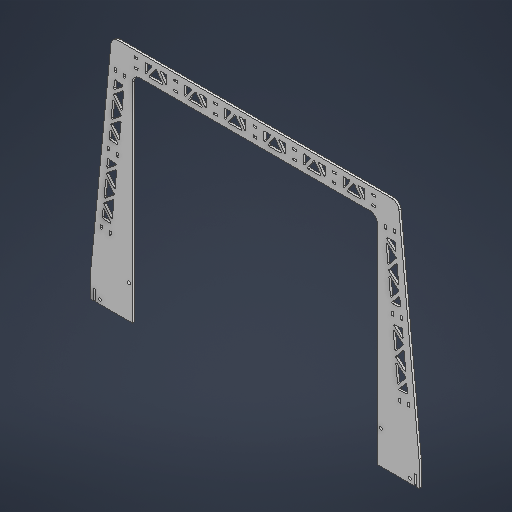
# Autodesk Inventor part: GateBrigeSideLessMaterial
Saved by Autodesk Inventor 2026 (Build 300175000, 175)
## iProperties
Created: 2025-03-30
Part Number: GateBrigeSideLessMaterial
Material: Všeobecné
Document SubType Name: Modeling
Designer: 42060
Density: 1 g/cm^3
Appearance: Výchozí
Author: 42060
Autodesk Inventor part; units mm, degrees
ref_plane "YZ Plane" through (0, 0, 0) normal (1, 0, 0) x (0, 1, 0)
ref_plane "XZ Plane" through (0, 0, 0) normal (0, 1, 0) x (-1, 0, 0)
ref_plane "XY Plane" through (0, 0, 0) normal (0, 0, 1) x (1, 0, 0)
sketch "Náčrt1" plane through (0, 0, 0) normal (0, 0, 1) x (1, 0, 0)
  line L0 (0, 0) -> (-160, 0)
  line L1 (-170, -10) -> (-170, -300)
  line L2 (-228, -300) -> (-228, -265.3)
  line L3 (-190.0475, 30) -> (0, 30)
  line L4 (0, 30) -> (0, 0)
  line L5 (-203.7, -249) -> (-170, -249)
  line L6 (-170, -249) -> (-170, -299)
  line L7 (-170, -299) -> (-220, -299)
  line L8 (-220, -299) -> (-220, -265.3)
  line L9 (-220, -265.3) -> (-203.7, -249)
  line L10 (-220, -299) -> (-170, -249) construction
  circle A0 centre (-215, -294) radius 2.1
  circle A1 centre (-175, -254) radius 2.1
  arc A2 (-160, 0) -> (-170, -10) centre (-160, -10) ccw
  line L11 (-200, 20.9734) -> (-228, -265.3)
  arc A3 (-190.0475, 30) -> (-200, 20.9734) centre (-190.0475, 20) ccw
  line L12 (-224, -300) -> (-224, -285)
  line L13 (-224, -285) -> (-221, -285)
  line L14 (-221, -285) -> (-221, -300)
  line L15 (-170, -300) -> (-221, -300)
  line L16 (-224, -300) -> (-228, -300)
  line L17 (0, 0) -> (160, 0)
  line L18 (170, -10) -> (170, -300)
  line L19 (228, -300) -> (228, -265.3)
  line L20 (190.0475, 30) -> (0, 30)
  line L21 (203.7, -249) -> (170, -249)
  line L22 (170, -249) -> (170, -299)
  line L23 (170, -299) -> (220, -299)
  line L24 (220, -299) -> (220, -265.3)
  line L25 (220, -265.3) -> (203.7, -249)
  line L26 (220, -299) -> (170, -249) construction
  circle A4 centre (215, -294) radius 2.1
  circle A5 centre (175, -254) radius 2.1
  arc A6 (170, -10) -> (160, 0) centre (160, -10) ccw
  line L27 (200, 20.9734) -> (228, -265.3)
  arc A7 (200, 20.9734) -> (190.0475, 30) centre (190.0475, 20) ccw
  line L28 (224, -300) -> (224, -285)
  line L29 (224, -285) -> (221, -285)
  line L30 (221, -285) -> (221, -300)
  line L31 (170, -300) -> (221, -300)
  line L32 (224, -300) -> (228, -300)
  line L33 (-36.6095, 9.0611) -> (-28.3278, 21.2788)
  line L34 (-26.6722, 21.2788) -> (-18.3905, 9.0611)
  line L35 (-19.2183, 7.5) -> (-35.7817, 7.5)
  line L36 (-21.6095, 20.9389) -> (-14.3278, 10.1964)
  line L37 (-12.5, 10.7575) -> (-12.5, 21.5)
  line L38 (-13.5, 22.5) -> (-20.7817, 22.5)
  line L39 (-33.3905, 20.9389) -> (-40.6722, 10.1964)
  line L40 (-42.5, 10.7575) -> (-42.5, 21.5)
  line L41 (-41.5, 22.5) -> (-34.2183, 22.5)
  line L42 (-55, 15) -> (0, 15) construction
  arc A8 (-41.5, 22.5) -> (-42.5, 21.5) centre (-41.5, 21.5) ccw
  arc A9 (-33.3905, 20.9389) -> (-34.2183, 22.5) centre (-34.2183, 21.5) ccw
  arc A10 (-42.5, 10.7575) -> (-40.6722, 10.1964) centre (-41.5, 10.7575) ccw
  arc A11 (-36.6095, 9.0611) -> (-35.7817, 7.5) centre (-35.7817, 8.5) ccw
  arc A12 (-19.2183, 7.5) -> (-18.3905, 9.0611) centre (-19.2183, 8.5) ccw
  arc A13 (-26.6722, 21.2788) -> (-28.3278, 21.2788) centre (-27.5, 20.7178) ccw
  arc A14 (-20.7817, 22.5) -> (-21.6095, 20.9389) centre (-20.7817, 21.5) ccw
  arc A15 (-12.5, 21.5) -> (-13.5, 22.5) centre (-13.5, 21.5) ccw
  arc A16 (-14.3278, 10.1964) -> (-12.5, 10.7575) centre (-13.5, 10.7575) ccw
  arc A17 (-81.6722, 21.2788) -> (-83.3278, 21.2788) centre (-82.5, 20.7178) ccw
  line L43 (-91.6095, 9.0611) -> (-83.3278, 21.2788)
  line L44 (-68.5, 22.5) -> (-75.7817, 22.5)
  arc A18 (-67.5, 21.5) -> (-68.5, 22.5) centre (-68.5, 21.5) ccw
  line L45 (-81.6722, 21.2788) -> (-73.3905, 9.0611)
  arc A19 (-74.2183, 7.5) -> (-73.3905, 9.0611) centre (-74.2183, 8.5) ccw
  line L46 (-76.6095, 20.9389) -> (-69.3278, 10.1964)
  line L47 (-74.2183, 7.5) -> (-90.7817, 7.5)
  arc A20 (-69.3278, 10.1964) -> (-67.5, 10.7575) centre (-68.5, 10.7575) ccw
  line L48 (-110, 15) -> (-55, 15) construction
  arc A21 (-96.5, 22.5) -> (-97.5, 21.5) centre (-96.5, 21.5) ccw
  arc A22 (-97.5, 10.7575) -> (-95.6722, 10.1964) centre (-96.5, 10.7575) ccw
  arc A23 (-91.6095, 9.0611) -> (-90.7817, 7.5) centre (-90.7817, 8.5) ccw
  arc A24 (-88.3905, 20.9389) -> (-89.2183, 22.5) centre (-89.2183, 21.5) ccw
  line L49 (-67.5, 10.7575) -> (-67.5, 21.5)
  arc A25 (-75.7817, 22.5) -> (-76.6095, 20.9389) centre (-75.7817, 21.5) ccw
  line L50 (-96.5, 22.5) -> (-89.2183, 22.5)
  line L51 (-88.3905, 20.9389) -> (-95.6722, 10.1964)
  line L52 (-97.5, 10.7575) -> (-97.5, 21.5)
  arc A26 (-136.6722, 21.2788) -> (-138.3278, 21.2788) centre (-137.5, 20.7178) ccw
  line L53 (-146.6095, 9.0611) -> (-138.3278, 21.2788)
  line L54 (-123.5, 22.5) -> (-130.7817, 22.5)
  arc A27 (-122.5, 21.5) -> (-123.5, 22.5) centre (-123.5, 21.5) ccw
  line L55 (-136.6722, 21.2788) -> (-128.3905, 9.0611)
  arc A28 (-129.2183, 7.5) -> (-128.3905, 9.0611) centre (-129.2183, 8.5) ccw
  line L56 (-131.6095, 20.9389) -> (-124.3278, 10.1964)
  line L57 (-129.2183, 7.5) -> (-145.7817, 7.5)
  arc A29 (-124.3278, 10.1964) -> (-122.5, 10.7575) centre (-123.5, 10.7575) ccw
  line L58 (-165, 15) -> (-110, 15) construction
  arc A30 (-151.5, 22.5) -> (-152.5, 21.5) centre (-151.5, 21.5) ccw
  arc A31 (-152.5, 10.7575) -> (-150.6722, 10.1964) centre (-151.5, 10.7575) ccw
  arc A32 (-146.6095, 9.0611) -> (-145.7817, 7.5) centre (-145.7817, 8.5) ccw
  arc A33 (-143.3905, 20.9389) -> (-144.2183, 22.5) centre (-144.2183, 21.5) ccw
  line L59 (-122.5, 10.7575) -> (-122.5, 21.5)
  arc A34 (-130.7817, 22.5) -> (-131.6095, 20.9389) centre (-130.7817, 21.5) ccw
  line L60 (-151.5, 22.5) -> (-144.2183, 22.5)
  line L61 (-143.3905, 20.9389) -> (-150.6722, 10.1964)
  line L62 (-152.5, 10.7575) -> (-152.5, 21.5)
  line L63 (-193.8722, -19.4692) -> (-183.9904, -20.4358)
  line L64 (-183.4529, -22.2036) -> (-194.3012, -31.1189)
  line L65 (-195.9313, -30.2489) -> (-194.9648, -20.3672)
  line L66 (-182.3734, -28.7035) -> (-184.5011, -50.4576)
  line L67 (-186.2689, -50.9951) -> (-196.0821, -39.0542)
  line L68 (-195.9444, -37.6468) -> (-184.0035, -27.8336)
  line L69 (-195.7348, -45.7768) -> (-185.9217, -57.7177)
  line L70 (-186.0594, -59.1252) -> (-198.0002, -68.9384)
  line L71 (-199.6304, -68.0685) -> (-197.5027, -46.3144)
  line L72 (-187.7026, -65.6531) -> (-199.6435, -75.4663)
  line L73 (-199.7812, -76.8738) -> (-189.968, -88.8147)
  line L74 (-188.2002, -88.2771) -> (-186.0724, -66.523)
  line L75 (-199.4339, -83.5964) -> (-190.5187, -94.4447)
  line L76 (-191.3886, -96.0748) -> (-201.2704, -95.1083)
  line L77 (-202.1683, -94.0157) -> (-201.2018, -84.1339)
  line L78 (-188.9313, -19.9525) -> (-188.0066, -10.4976) construction
  arc A35 (-193.8722, -19.4692) -> (-194.9648, -20.3672) centre (-193.9696, -20.4645) ccw
  arc A36 (-183.4529, -22.2036) -> (-183.9904, -20.4358) centre (-184.0878, -21.431) ccw
  arc A37 (-195.9313, -30.2489) -> (-194.3012, -31.1189) centre (-194.9361, -30.3463) ccw
  arc A38 (-195.9444, -37.6468) -> (-196.0821, -39.0542) centre (-195.3095, -38.4193) ccw
  arc A39 (-186.2689, -50.9951) -> (-184.5011, -50.4576) centre (-185.4963, -50.3602) ccw
  arc A40 (-182.3734, -28.7035) -> (-184.0035, -27.8336) centre (-183.3686, -28.6062) ccw
  arc A41 (-195.7348, -45.7768) -> (-197.5027, -46.3144) centre (-196.5074, -46.4117) ccw
  arc A42 (-186.0594, -59.1252) -> (-185.9217, -57.7177) centre (-186.6943, -58.3526) ccw
  arc A43 (-199.6304, -68.0685) -> (-198.0002, -68.9384) centre (-198.6352, -68.1658) ccw
  arc A44 (-199.6435, -75.4663) -> (-199.7812, -76.8738) centre (-199.0086, -76.2389) ccw
  arc A45 (-189.968, -88.8147) -> (-188.2002, -88.2771) centre (-189.1954, -88.1798) ccw
  arc A46 (-186.0724, -66.523) -> (-187.7026, -65.6531) centre (-187.0677, -66.4257) ccw
  arc A47 (-199.4339, -83.5964) -> (-201.2018, -84.1339) centre (-200.2065, -84.2313) ccw
  arc A48 (-202.1683, -94.0157) -> (-201.2704, -95.1083) centre (-201.173, -94.1131) ccw
  arc A49 (-191.3886, -96.0748) -> (-190.5187, -94.4447) centre (-191.2912, -95.0796) ccw
  arc A50 (-211.9027, -193.5408) -> (-211.0048, -194.6334) centre (-210.9074, -193.6381) ccw
  line L79 (-201.123, -195.5999) -> (-211.0048, -194.6334)
  arc A51 (-201.123, -195.5999) -> (-200.2531, -193.9697) centre (-201.0257, -194.6047) ccw
  arc A52 (-199.7024, -188.3398) -> (-197.9346, -187.8022) centre (-198.9298, -187.7048) ccw
  line L80 (-209.1683, -183.1214) -> (-200.2531, -193.9697)
  line L81 (-211.9027, -193.5408) -> (-210.9362, -183.659)
  arc A53 (-209.1683, -183.1214) -> (-210.9362, -183.659) centre (-209.9409, -183.7564) ccw
  line L82 (-197.437, -165.1782) -> (-209.3779, -174.9914)
  line L83 (-209.5156, -176.3989) -> (-199.7024, -188.3398)
  line L84 (-197.9346, -187.8022) -> (-195.8068, -166.0481)
  arc A54 (-209.3779, -174.9914) -> (-209.5156, -176.3989) centre (-208.743, -175.7639) ccw
  arc A55 (-209.3648, -167.5935) -> (-207.7347, -168.4635) centre (-208.3696, -167.6909) ccw
  arc A56 (-195.8068, -166.0481) -> (-197.437, -165.1782) centre (-196.8021, -165.9508) ccw
  line L85 (-205.4693, -145.3019) -> (-195.6561, -157.2428)
  arc A57 (-195.7938, -158.6503) -> (-195.6561, -157.2428) centre (-196.4287, -157.8777) ccw
  line L86 (-209.3648, -167.5935) -> (-207.2371, -145.8395)
  line L87 (-195.7938, -158.6503) -> (-207.7347, -168.4635)
  arc A58 (-196.0033, -150.5202) -> (-194.2355, -149.9827) centre (-195.2308, -149.8853) ccw
  arc A59 (-205.4693, -145.3019) -> (-207.2371, -145.8395) centre (-206.2418, -145.9368) ccw
  line L88 (-196.0033, -150.5202) -> (-205.8165, -138.5793)
  arc A60 (-205.6788, -137.1718) -> (-205.8165, -138.5793) centre (-205.0439, -137.9444) ccw
  arc A61 (-205.6657, -129.774) -> (-204.0356, -130.6439) centre (-204.6705, -129.8714) ccw
  line L89 (-192.1078, -128.2286) -> (-194.2355, -149.9827)
  line L90 (-205.6788, -137.1718) -> (-193.7379, -127.3587)
  arc A62 (-192.1078, -128.2286) -> (-193.7379, -127.3587) centre (-193.103, -128.1312) ccw
  arc A63 (-193.1873, -121.7287) -> (-193.7248, -119.9608) centre (-193.8222, -120.9561) ccw
  line L91 (-198.6657, -119.4776) -> (-197.741, -110.0227) construction
  line L92 (-203.6066, -118.9943) -> (-193.7248, -119.9608)
  arc A64 (-203.6066, -118.9943) -> (-204.6992, -119.8922) centre (-203.704, -119.9896) ccw
  line L93 (-193.1873, -121.7287) -> (-204.0356, -130.6439)
  line L94 (-205.6657, -129.774) -> (-204.6992, -119.8922)
  line L95 (36.6095, 9.0611) -> (28.3278, 21.2788)
  line L96 (26.6722, 21.2788) -> (18.3905, 9.0611)
  line L97 (19.2183, 7.5) -> (35.7817, 7.5)
  line L98 (21.6095, 20.9389) -> (14.3278, 10.1964)
  line L99 (12.5, 10.7575) -> (12.5, 21.5)
  line L100 (13.5, 22.5) -> (20.7817, 22.5)
  line L101 (33.3905, 20.9389) -> (40.6722, 10.1964)
  line L102 (42.5, 10.7575) -> (42.5, 21.5)
  line L103 (41.5, 22.5) -> (34.2183, 22.5)
  line L104 (55, 15) -> (0, 15) construction
  arc A65 (42.5, 21.5) -> (41.5, 22.5) centre (41.5, 21.5) ccw
  arc A66 (34.2183, 22.5) -> (33.3905, 20.9389) centre (34.2183, 21.5) ccw
  arc A67 (40.6722, 10.1964) -> (42.5, 10.7575) centre (41.5, 10.7575) ccw
  arc A68 (35.7817, 7.5) -> (36.6095, 9.0611) centre (35.7817, 8.5) ccw
  arc A69 (18.3905, 9.0611) -> (19.2183, 7.5) centre (19.2183, 8.5) ccw
  arc A70 (28.3278, 21.2788) -> (26.6722, 21.2788) centre (27.5, 20.7178) ccw
  arc A71 (21.6095, 20.9389) -> (20.7817, 22.5) centre (20.7817, 21.5) ccw
  arc A72 (13.5, 22.5) -> (12.5, 21.5) centre (13.5, 21.5) ccw
  arc A73 (12.5, 10.7575) -> (14.3278, 10.1964) centre (13.5, 10.7575) ccw
  line L105 (67.5, 10.7575) -> (67.5, 21.5)
  line L106 (96.5, 22.5) -> (89.2183, 22.5)
  arc A74 (97.5, 21.5) -> (96.5, 22.5) centre (96.5, 21.5) ccw
  line L107 (97.5, 10.7575) -> (97.5, 21.5)
  arc A75 (95.6722, 10.1964) -> (97.5, 10.7575) centre (96.5, 10.7575) ccw
  arc A76 (67.5, 10.7575) -> (69.3278, 10.1964) centre (68.5, 10.7575) ccw
  arc A77 (68.5, 22.5) -> (67.5, 21.5) centre (68.5, 21.5) ccw
  arc A78 (89.2183, 22.5) -> (88.3905, 20.9389) centre (89.2183, 21.5) ccw
  arc A79 (83.3278, 21.2788) -> (81.6722, 21.2788) centre (82.5, 20.7178) ccw
  line L108 (88.3905, 20.9389) -> (95.6722, 10.1964)
  line L109 (91.6095, 9.0611) -> (83.3278, 21.2788)
  arc A80 (76.6095, 20.9389) -> (75.7817, 22.5) centre (75.7817, 21.5) ccw
  arc A81 (90.7817, 7.5) -> (91.6095, 9.0611) centre (90.7817, 8.5) ccw
  line L110 (110, 15) -> (55, 15) construction
  line L111 (68.5, 22.5) -> (75.7817, 22.5)
  line L112 (76.6095, 20.9389) -> (69.3278, 10.1964)
  line L113 (81.6722, 21.2788) -> (73.3905, 9.0611)
  arc A82 (73.3905, 9.0611) -> (74.2183, 7.5) centre (74.2183, 8.5) ccw
  line L114 (74.2183, 7.5) -> (90.7817, 7.5)
  line L115 (122.5, 10.7575) -> (122.5, 21.5)
  line L116 (151.5, 22.5) -> (144.2183, 22.5)
  arc A83 (152.5, 21.5) -> (151.5, 22.5) centre (151.5, 21.5) ccw
  line L117 (152.5, 10.7575) -> (152.5, 21.5)
  arc A84 (150.6722, 10.1964) -> (152.5, 10.7575) centre (151.5, 10.7575) ccw
  arc A85 (122.5, 10.7575) -> (124.3278, 10.1964) centre (123.5, 10.7575) ccw
  arc A86 (123.5, 22.5) -> (122.5, 21.5) centre (123.5, 21.5) ccw
  arc A87 (144.2183, 22.5) -> (143.3905, 20.9389) centre (144.2183, 21.5) ccw
  arc A88 (138.3278, 21.2788) -> (136.6722, 21.2788) centre (137.5, 20.7178) ccw
  line L118 (143.3905, 20.9389) -> (150.6722, 10.1964)
  line L119 (146.6095, 9.0611) -> (138.3278, 21.2788)
  arc A89 (131.6095, 20.9389) -> (130.7817, 22.5) centre (130.7817, 21.5) ccw
  arc A90 (145.7817, 7.5) -> (146.6095, 9.0611) centre (145.7817, 8.5) ccw
  line L120 (165, 15) -> (110, 15) construction
  line L121 (123.5, 22.5) -> (130.7817, 22.5)
  line L122 (131.6095, 20.9389) -> (124.3278, 10.1964)
  line L123 (136.6722, 21.2788) -> (128.3905, 9.0611)
  arc A91 (128.3905, 9.0611) -> (129.2183, 7.5) centre (129.2183, 8.5) ccw
  line L124 (129.2183, 7.5) -> (145.7817, 7.5)
  line L125 (193.8722, -19.4692) -> (183.9904, -20.4358)
  line L126 (183.4529, -22.2036) -> (194.3012, -31.1189)
  line L127 (195.9313, -30.2489) -> (194.9648, -20.3672)
  line L128 (182.3734, -28.7035) -> (184.5011, -50.4576)
  line L129 (186.2689, -50.9951) -> (196.0821, -39.0542)
  line L130 (195.9444, -37.6468) -> (184.0035, -27.8336)
  line L131 (195.7348, -45.7768) -> (185.9217, -57.7177)
  line L132 (186.0594, -59.1252) -> (198.0002, -68.9384)
  line L133 (199.6304, -68.0685) -> (197.5027, -46.3144)
  line L134 (187.7026, -65.6531) -> (199.6435, -75.4663)
  line L135 (199.7812, -76.8738) -> (189.968, -88.8147)
  line L136 (188.2002, -88.2771) -> (186.0724, -66.523)
  line L137 (199.4339, -83.5964) -> (190.5187, -94.4447)
  line L138 (191.3886, -96.0748) -> (201.2704, -95.1083)
  line L139 (202.1683, -94.0157) -> (201.2018, -84.1339)
  arc A92 (194.9648, -20.3672) -> (193.8722, -19.4692) centre (193.9696, -20.4645) ccw
  arc A93 (183.9904, -20.4358) -> (183.4529, -22.2036) centre (184.0878, -21.431) ccw
  arc A94 (194.3012, -31.1189) -> (195.9313, -30.2489) centre (194.9361, -30.3463) ccw
  arc A95 (196.0821, -39.0542) -> (195.9444, -37.6468) centre (195.3095, -38.4193) ccw
  arc A96 (184.5011, -50.4576) -> (186.2689, -50.9951) centre (185.4963, -50.3602) ccw
  arc A97 (184.0035, -27.8336) -> (182.3734, -28.7035) centre (183.3686, -28.6062) ccw
  arc A98 (197.5027, -46.3144) -> (195.7348, -45.7768) centre (196.5074, -46.4117) ccw
  arc A99 (185.9217, -57.7177) -> (186.0594, -59.1252) centre (186.6943, -58.3526) ccw
  arc A100 (198.0002, -68.9384) -> (199.6304, -68.0685) centre (198.6352, -68.1658) ccw
  arc A101 (199.7812, -76.8738) -> (199.6435, -75.4663) centre (199.0086, -76.2389) ccw
  arc A102 (188.2002, -88.2771) -> (189.968, -88.8147) centre (189.1954, -88.1798) ccw
  arc A103 (187.7026, -65.6531) -> (186.0724, -66.523) centre (187.0677, -66.4257) ccw
  arc A104 (201.2018, -84.1339) -> (199.4339, -83.5964) centre (200.2065, -84.2313) ccw
  arc A105 (201.2704, -95.1083) -> (202.1683, -94.0157) centre (201.173, -94.1131) ccw
  arc A106 (190.5187, -94.4447) -> (191.3886, -96.0748) centre (191.2912, -95.0796) ccw
  arc A107 (193.7248, -119.9608) -> (193.1873, -121.7287) centre (193.8222, -120.9561) ccw
  arc A108 (193.7379, -127.3587) -> (192.1078, -128.2286) centre (193.103, -128.1312) ccw
  line L140 (203.6066, -118.9943) -> (193.7248, -119.9608)
  line L141 (193.1873, -121.7287) -> (204.0356, -130.6439)
  line L142 (205.6657, -129.774) -> (204.6992, -119.8922)
  line L143 (205.6788, -137.1718) -> (193.7379, -127.3587)
  arc A109 (204.6992, -119.8922) -> (203.6066, -118.9943) centre (203.704, -119.9896) ccw
  arc A110 (204.0356, -130.6439) -> (205.6657, -129.774) centre (204.6705, -129.8714) ccw
  line L144 (192.1078, -128.2286) -> (194.2355, -149.9827)
  arc A111 (207.2371, -145.8395) -> (205.4693, -145.3019) centre (206.2418, -145.9368) ccw
  line L145 (196.0033, -150.5202) -> (205.8165, -138.5793)
  arc A112 (205.8165, -138.5793) -> (205.6788, -137.1718) centre (205.0439, -137.9444) ccw
  arc A113 (194.2355, -149.9827) -> (196.0033, -150.5202) centre (195.2308, -149.8853) ccw
  line L146 (205.4693, -145.3019) -> (195.6561, -157.2428)
  arc A114 (195.6561, -157.2428) -> (195.7938, -158.6503) centre (196.4287, -157.8777) ccw
  arc A115 (197.437, -165.1782) -> (195.8068, -166.0481) centre (196.8021, -165.9508) ccw
  line L147 (195.7938, -158.6503) -> (207.7347, -168.4635)
  arc A116 (207.7347, -168.4635) -> (209.3648, -167.5935) centre (208.3696, -167.6909) ccw
  line L148 (209.3648, -167.5935) -> (207.2371, -145.8395)
  arc A117 (200.2531, -193.9697) -> (201.123, -195.5999) centre (201.0257, -194.6047) ccw
  arc A118 (211.0048, -194.6334) -> (211.9027, -193.5408) centre (210.9074, -193.6381) ccw
  arc A119 (197.9346, -187.8022) -> (199.7024, -188.3398) centre (198.9298, -187.7048) ccw
  line L149 (211.9027, -193.5408) -> (210.9362, -183.659)
  line L150 (209.1683, -183.1214) -> (200.2531, -193.9697)
  arc A120 (210.9362, -183.659) -> (209.1683, -183.1214) centre (209.9409, -183.7564) ccw
  line L151 (209.5156, -176.3989) -> (199.7024, -188.3398)
  arc A121 (209.5156, -176.3989) -> (209.3779, -174.9914) centre (208.743, -175.7639) ccw
  line L152 (197.9346, -187.8022) -> (195.8068, -166.0481)
  line L153 (197.437, -165.1782) -> (209.3779, -174.9914)
  line L154 (201.123, -195.5999) -> (211.0048, -194.6334)
  line L155 (-2.5, 10) -> (2.5, 10)
  line L156 (2.5, 10) -> (2.5, 7.5)
  line L157 (2.5, 7.5) -> (-2.5, 7.5)
  line L158 (-2.5, 7.5) -> (-2.5, 10)
  line L159 (-2.5, 22.5) -> (2.5, 22.5)
  line L160 (2.5, 22.5) -> (2.5, 20)
  line L161 (2.5, 20) -> (-2.5, 20)
  line L162 (-2.5, 20) -> (-2.5, 22.5)
  line L163 (0, 20) -> (0, 10) construction
  line L164 (-42.5, 10.7575) -> (-42.5, 7.5) construction
  line L165 (-42.5, 7.5) -> (-40.6722, 10.1964) construction
  line L166 (-27.5, 22.5) -> (-27.5, 7.5) construction
  line L167 (-52.5, 10) -> (-52.5, 7.5)
  line L168 (-57.5, 10) -> (-52.5, 10)
  line L169 (-52.5, 7.5) -> (-57.5, 7.5)
  line L170 (-57.5, 7.5) -> (-57.5, 10)
  line L171 (-57.5, 22.5) -> (-52.5, 22.5)
  line L172 (-52.5, 20) -> (-57.5, 20)
  line L173 (-57.5, 20) -> (-57.5, 22.5)
  line L174 (-52.5, 22.5) -> (-52.5, 20)
  line L175 (-107.5, 10) -> (-107.5, 7.5)
  line L176 (-112.5, 10) -> (-107.5, 10)
  line L177 (-107.5, 7.5) -> (-112.5, 7.5)
  line L178 (-112.5, 7.5) -> (-112.5, 10)
  line L179 (-112.5, 22.5) -> (-107.5, 22.5)
  line L180 (-107.5, 20) -> (-112.5, 20)
  line L181 (-112.5, 20) -> (-112.5, 22.5)
  line L182 (-107.5, 22.5) -> (-107.5, 20)
  line L183 (-162.5, 10) -> (-162.5, 7.5)
  line L184 (-167.5, 10) -> (-162.5, 10)
  line L185 (-162.5, 7.5) -> (-167.5, 7.5)
  line L186 (-167.5, 7.5) -> (-167.5, 10)
  line L187 (-167.5, 22.5) -> (-162.5, 22.5)
  line L188 (-162.5, 20) -> (-167.5, 20)
  line L189 (-167.5, 20) -> (-167.5, 22.5)
  line L190 (-162.5, 22.5) -> (-162.5, 20)
  line L191 (52.5, 20) -> (52.5, 22.5)
  line L192 (57.5, 20) -> (52.5, 20)
  line L193 (57.5, 22.5) -> (57.5, 20)
  line L194 (52.5, 22.5) -> (57.5, 22.5)
  line L195 (57.5, 10) -> (57.5, 7.5)
  line L196 (52.5, 10) -> (57.5, 10)
  line L197 (57.5, 7.5) -> (52.5, 7.5)
  line L198 (52.5, 7.5) -> (52.5, 10)
  line L199 (107.5, 20) -> (107.5, 22.5)
  line L200 (112.5, 20) -> (107.5, 20)
  line L201 (112.5, 22.5) -> (112.5, 20)
  line L202 (107.5, 22.5) -> (112.5, 22.5)
  line L203 (112.5, 10) -> (112.5, 7.5)
  line L204 (107.5, 10) -> (112.5, 10)
  line L205 (112.5, 7.5) -> (107.5, 7.5)
  line L206 (107.5, 7.5) -> (107.5, 10)
  line L207 (162.5, 20) -> (162.5, 22.5)
  line L208 (167.5, 20) -> (162.5, 20)
  line L209 (167.5, 22.5) -> (167.5, 20)
  line L210 (162.5, 22.5) -> (167.5, 22.5)
  line L211 (167.5, 10) -> (167.5, 7.5)
  line L212 (162.5, 10) -> (167.5, 10)
  line L213 (167.5, 7.5) -> (162.5, 7.5)
  line L214 (162.5, 7.5) -> (162.5, 10)
  line L215 (-194.9842, -4.7913) -> (-192.4961, -5.0347)
  line L216 (-192.4961, -5.0347) -> (-192.9828, -10.0109)
  line L217 (-192.9828, -10.0109) -> (-195.4709, -9.7675)
  line L218 (-195.4709, -9.7675) -> (-194.9842, -4.7913)
  line L219 (-182.5436, -6.0081) -> (-180.0555, -6.2515)
  line L220 (-180.0555, -6.2515) -> (-180.5422, -11.2277)
  line L221 (-180.5422, -11.2277) -> (-183.0303, -10.9843)
  line L222 (-183.0303, -10.9843) -> (-182.5436, -6.0081)
  line L223 (-192.9828, -10.0109) -> (-183.0303, -10.9843) construction
  line L224 (-205.2054, -109.2926) -> (-204.7186, -104.3164)
  line L225 (-202.2305, -104.5597) -> (-202.7172, -109.536)
  line L226 (-202.7172, -109.536) -> (-205.2054, -109.2926)
  line L227 (-204.7186, -104.3164) -> (-202.2305, -104.5597)
  line L228 (-192.7647, -110.5094) -> (-192.278, -105.5332)
  line L229 (-190.2766, -110.7528) -> (-192.7647, -110.5094)
  line L230 (-189.7899, -105.7765) -> (-190.2766, -110.7528)
  line L231 (-192.278, -105.5332) -> (-189.7899, -105.7765)
  line L232 (-202.7172, -109.536) -> (-192.7647, -110.5094) construction
  line L233 (-202.2305, -104.5597) -> (-192.278, -105.5332) construction
  line L234 (-197.3029, -105.5441) -> (-196.3295, -95.5916) construction
  line L235 (-214.9398, -208.8177) -> (-214.453, -203.8414)
  line L236 (-211.9649, -204.0848) -> (-212.4516, -209.0611)
  line L237 (-212.4516, -209.0611) -> (-214.9398, -208.8177)
  line L238 (-214.453, -203.8414) -> (-211.9649, -204.0848)
  line L239 (-202.4991, -210.0345) -> (-202.0124, -205.0582)
  line L240 (-200.011, -210.2779) -> (-202.4991, -210.0345)
  line L241 (-199.5243, -205.3016) -> (-200.011, -210.2779)
  line L242 (-202.0124, -205.0582) -> (-199.5243, -205.3016)
  line L243 (-212.4516, -209.0611) -> (-202.4991, -210.0345) construction
  line L244 (194.9842, -4.7913) -> (192.4961, -5.0347)
  line L245 (192.4961, -5.0347) -> (192.9828, -10.0109)
  line L246 (192.9828, -10.0109) -> (195.4709, -9.7675)
  line L247 (195.4709, -9.7675) -> (194.9842, -4.7913)
  line L248 (182.5436, -6.0081) -> (180.0555, -6.2515)
  line L249 (180.0555, -6.2515) -> (180.5422, -11.2277)
  line L250 (180.5422, -11.2277) -> (183.0303, -10.9843)
  line L251 (183.0303, -10.9843) -> (182.5436, -6.0081)
  line L252 (205.2054, -109.2926) -> (204.7186, -104.3164)
  line L253 (202.2305, -104.5597) -> (202.7172, -109.536)
  line L254 (202.7172, -109.536) -> (205.2054, -109.2926)
  line L255 (204.7186, -104.3164) -> (202.2305, -104.5597)
  line L256 (192.7647, -110.5094) -> (192.278, -105.5332)
  line L257 (190.2766, -110.7528) -> (192.7647, -110.5094)
  line L258 (189.7899, -105.7765) -> (190.2766, -110.7528)
  line L259 (192.278, -105.5332) -> (189.7899, -105.7765)
  line L260 (214.9398, -208.8177) -> (214.453, -203.8414)
  line L261 (211.9649, -204.0848) -> (212.4516, -209.0611)
  line L262 (212.4516, -209.0611) -> (214.9398, -208.8177)
  line L263 (214.453, -203.8414) -> (211.9649, -204.0848)
  line L264 (202.4991, -210.0345) -> (202.0124, -205.0582)
  line L265 (200.011, -210.2779) -> (202.4991, -210.0345)
  line L266 (199.5243, -205.3016) -> (200.011, -210.2779)
  line L267 (202.0124, -205.0582) -> (199.5243, -205.3016)
  line L268 (-188.0066, -10.4976) -> (-187.9579, -10) construction
  point P0 (-12.5, 7.5)
  point P1 (-32.3323, 22.5)
  point P2 (-42.5, 22.5)
  point P3 (-27.5, 15)
  point P4 (-12.5, 16.1288)
  point P5 (-82.5, 22.5)
  point P6 (-82.5, 15)
  point P7 (-82.5, 7.5)
  point P8 (-87.3323, 22.5)
  point P9 (-97.5, 22.5)
  point P10 (-67.5, 7.5)
  point P11 (-67.5, 16.1288)
  point P12 (-137.5, 22.5)
  point P13 (-137.5, 15)
  point P14 (-137.5, 7.5)
  point P15 (-142.3323, 22.5)
  point P16 (-152.5, 22.5)
  point P17 (-122.5, 7.5)
  point P18 (-122.5, 16.1288)
  point P19 (-194.8675, -19.3719)
  point P20 (-181.5877, -20.6708)
  point P21 (-196.1663, -32.6517)
  point P22 (-182.1384, -26.3008)
  point P23 (-184.7361, -52.8603)
  point P24 (-196.717, -38.2817)
  point P25 (-197.2677, -43.9117)
  point P26 (-185.2868, -58.4903)
  point P27 (-199.8654, -70.4712)
  point P28 (-185.8374, -64.1203)
  point P29 (-200.4161, -76.1012)
  point P30 (-188.4352, -90.6798)
  point P31 (-200.9667, -81.7312)
  point P32 (-188.9858, -96.3098)
  point P33 (-202.2656, -95.011)
  point P34 (-212, -194.536)
  point P35 (-198.7203, -195.8349)
  point P36 (-198.1696, -190.2049)
  point P37 (-210.7012, -181.2563)
  point P38 (-210.1505, -175.6263)
  point P39 (-209.5998, -169.9963)
  point P40 (-195.5718, -163.6454)
  point P41 (-195.0212, -158.0154)
  point P42 (-194.4705, -152.3854)
  point P43 (-207.0021, -143.4367)
  point P44 (-206.4514, -137.8067)
  point P45 (-205.9008, -132.1768)
  point P46 (-191.8728, -125.8258)
  point P47 (-191.3221, -120.1959)
  point P48 (-204.6019, -118.897)
  point P49 (27.5, 22.5)
  point P50 (12.5, 7.5)
  point P51 (32.3323, 22.5)
  point P52 (42.5, 22.5)
  point P53 (27.5, 7.5)
  point P54 (27.5, 15)
  point P55 (12.5, 16.1288)
  point P56 (67.5, 7.5)
  point P57 (67.5, 16.1288)
  point P58 (82.5, 22.5)
  point P59 (87.3323, 22.5)
  point P60 (97.5, 22.5)
  point P61 (82.5, 15)
  point P62 (82.5, 7.5)
  point P63 (122.5, 7.5)
  point P64 (122.5, 16.1288)
  point P65 (137.5, 22.5)
  point P66 (142.3323, 22.5)
  point P67 (152.5, 22.5)
  point P68 (137.5, 15)
  point P69 (137.5, 7.5)
  point P70 (194.8675, -19.3719)
  point P71 (181.5877, -20.6708)
  point P72 (196.1663, -32.6517)
  point P73 (182.1384, -26.3008)
  point P74 (184.7361, -52.8603)
  point P75 (196.717, -38.2817)
  point P76 (197.2677, -43.9117)
  point P77 (185.2868, -58.4903)
  point P78 (199.8654, -70.4712)
  point P79 (185.8374, -64.1203)
  point P80 (200.4161, -76.1012)
  point P81 (188.4352, -90.6798)
  point P82 (200.9667, -81.7312)
  point P83 (188.9858, -96.3098)
  point P84 (202.2656, -95.011)
  point P85 (188.9313, -19.9525)
  point P86 (191.3221, -120.1959)
  point P87 (191.8728, -125.8258)
  point P88 (198.6657, -119.4776)
  point P89 (204.6019, -118.897)
  point P90 (205.9008, -132.1768)
  point P91 (206.4514, -137.8067)
  point P92 (194.4705, -152.3854)
  point P93 (207.0021, -143.4367)
  point P94 (195.0212, -158.0154)
  point P95 (195.5718, -163.6454)
  point P96 (209.5998, -169.9963)
  point P97 (212, -194.536)
  point P98 (198.7203, -195.8349)
  point P99 (198.1696, -190.2049)
  point P100 (210.1505, -175.6263)
  point P101 (210.7012, -181.2563)
  point P102 (0, 15)
  point P103 (-27.5, 15)
  point P104 (-55, 10)
  point P105 (-55, 20)
  point P106 (-110, 10)
  point P107 (-110, 20)
  point P108 (-165, 10)
  point P109 (-165, 20)
  point P110 (55, 20)
  point P111 (55, 10)
  point P112 (110, 20)
  point P113 (110, 10)
  point P114 (165, 20)
  point P115 (165, 10)
  point P116 (-207.4754, -209.5478)
  point P117 (-197.2542, -105.0465)
  dimension "d0" = 50
  dimension "d1" = 50
  dimension "d3" = 33.7
  dimension "d4" = 45
  dimension "d5" = 0
  dimension "d6" = 4.2
  dimension "d7" = 5
  dimension "d8" = 5
  dimension "d10" = 170
  dimension "d12" = 30
  dimension "d14" = 10
  dimension "d16" = 15
  dimension "d17" = 1
  dimension "d18" = 3
  dimension "d19" = 1
  dimension "d20" = 4
  dimension "d21" = 300
  dimension "d22" = 30
  dimension "d46" = 4
  dimension "d47" = 4
  dimension "d50" = 15
  dimension "d51" = 30
  dimension "d52" = 1
  dimension "d55" = 55
  dimension "d63" = 4
  dimension "d64" = 4
  dimension "d65" = 4
  dimension "d66" = 4
  dimension "d67" = 1
  dimension "d70" = 100
  dimension "d77" = 55
  dimension "d84" = 100
  dimension "d91" = 2.5
  dimension "d92" = 5
  dimension "d93" = 15
  dimension "d96" = 55
  dimension "d103" = 55
  dimension "d108" = 5
  dimension "d109" = 2.5
  dimension "d110" = 7.5
  dimension "d111" = 15
  dimension "d115" = 100
  dimension "d123" = 0.5
  dimension "d124" = 0.5
  dimension "d125" = 10
  dimension "d126" = 10
  constraints: 538 end point, 236 point on circle, 227 point on line, 141 symmetric about line, 122 centre point, 52 tangent, 24 equal radius, 24 perpendicular, 20 parallel, 12 midpoint, 11 collinear, 10 coincident, 10 horizontal, 5 equal length, 4 horizontal alignment, 4 vertical alignment, 2 vertical, 579 other
  measures "d0" distance of L5.end L6.end
  measures "d1" distance of L6.end L7.end
  measures "d3" distance of L5.start L5.end
  measures "d4" angle of L5 L9
  measures "d5" distance between parallel lines of L1 L6
  measures "d6" diameter of A1
  measures "d7" distance from line of L5 A1.centre
  measures "d8" distance from line of L7 A0.centre
  measures "d10" distance between parallel lines of L1 L4
  measures "d12" distance between parallel lines of L0 L3
  measures "d14" radius of A3
  measures "d16" distance between parallel lines of L16 L13
  measures "d17" distance between parallel lines of L7 L15
  measures "d18" distance between parallel lines of L14 L12
  measures "d19" distance between parallel lines of L8 L14
  measures "d20" distance between parallel lines of L12 L2
  measures "d21" distance between parallel lines of L15 L0
  measures "d22" distance from line of L11.start L1
  measures "d46" distance between parallel lines of L33 L39
  measures "d47" distance between parallel lines of L36 L34
  measures "d50" distance from line of L35 L166.start
  measures "d51" distance between parallel lines of L37 L40
  measures "d52" radius of A8
  measures "d55" distance of L166.start point (-82.5, 22.5)
  measures "d63" distance between parallel lines of L68 L64
  measures "d64" distance between parallel lines of L69 L67
  measures "d65" distance between parallel lines of L72 L70
  measures "d66" distance between parallel lines of L73 L75
  measures "d67" radius of A35
  measures "d70" distance of point (-202.266, -95.011) point (-212, -194.536)
  measures "d77" distance of point (12.5, 7.5) point (67.5, 7.5)
  measures "d84" distance of point (181.588, -20.671) point (191.322, -120.196)
  measures "d91" distance of L159.end L160.end
  measures "d92" distance of L159.start L159.end
  measures "d93" distance between parallel lines of L157 L159
  measures "d96" distance of L155.end L167.start
  measures "d103" distance of L159.start L191.end
  measures "d108" distance of L217.end L215.start
  measures "d109" distance of L215.start L215.end
  measures "d110" distance between parallel lines of L11 L218
  measures "d111" distance between parallel lines of L220 L218
  measures "d115" distance of L217.end L224.start
  measures "d123" distance of L268.start L268.end
  measures "d124" distance from line of L234.start L233
  measures "d125" distance of L78.start L268.end
  measures "d126" distance of L234.start L234.end
extrude "Vysunutí1" add sketch "Náčrt1" along normal blind 3 contours L0 A2 L1 L5 L9 L8 L7 L15 L14 L13 L12 L16 L2 L11 A3 L3 L4 L159 L162 L161 L155 L158 L157 | L4 L157 L156 L155 L161 L160 L159 L20 A7 L27 L19 L32 L28 L29 L30 L31 L18 L23 L24 L25 L21 A6 L17 | L1 L7 L8 L9 L5 | L21 L25 L24 L23 L18
equation "\"d44\" = d18"
